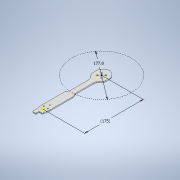
# Autodesk Inventor part: Kauri arm long
Saved by Autodesk Inventor 2020 (Build 240168000, 168)
## iProperties
Created: 2022-04-26
Part Number: Kauri arm long
Material: Generic
Document SubType Name: Modeling
Designer: Steve3
Density: 1 g/cm^3
Appearance: Default
Mass: 28.618 g
Surface Area: 128.182 cm^2
Volume: 28.618 cm^3
Sending System: Autodesk Inventor 2020
Preprocessor: ST-DEVELOPER v18
Title: Y:\Street League\Frames\Kauri\AAA LeadFingers version 2\github files\Kauri arm.stp
Author: Steven
Autodesk Inventor part; units mm, degrees
ref_plane "YZ Plane" through (0, 0, 0) normal (1, 0, 0) x (0, 1, 0)
ref_plane "XZ Plane" through (0, 0, 0) normal (0, 1, 0) x (-1, 0, 0)
ref_plane "XY Plane" through (0, 0, 0) normal (0, 0, 1) x (1, 0, 0)
sketch "Sketch3" plane through (0, 0, 0) normal (0, 1, 0) x (-1, 0, 0)
  line L0 (6.6262, -36.1747) -> (16.6262, -27.3275)
  arc A0 (16.6262, -27.3275) -> (20, -19.8379) centre (10, -19.8379) ccw
  line L1 (20, -19.8379) -> (20, -7.6759)
  arc A1 (20, -7.6759) -> (18, -1.6759) centre (10, -7.6759) ccw
  line L2 (18, -1.6759) -> (14.5, 2.9908)
  arc A2 (12.5, 8.9908) -> (14.5, 2.9908) centre (22.5, 8.9908) ccw
  arc A3 (-14.5, 2.9908) -> (-12.5, 8.9908) centre (-22.5, 8.9908) ccw
  line L3 (-14.5, 2.9908) -> (-18, -1.6759)
  arc A4 (-18, -1.6759) -> (-20, -7.6759) centre (-10, -7.6759) ccw
  line L4 (-20, -7.6759) -> (-20, -19.8379)
  arc A5 (-20, -19.8379) -> (-16.6262, -27.3275) centre (-10, -19.8379) ccw
  line L5 (-16.6262, -27.3275) -> (-6.6262, -36.1747)
  arc A6 (-6.6262, -36.1747) -> (6.6262, -36.1747) centre (0, -28.6852) ccw
  line L6 (-7.8135, -19.9641) -> (-6.7529, -18.9034)
  arc A7 (-4.5608, -21.0955) -> (-6.7529, -18.9034) centre (-5.6569, -19.9994) ccw
  line L7 (-4.5608, -21.0955) -> (-5.6215, -22.1561)
  arc A8 (-7.8135, -19.9641) -> (-5.6215, -22.1561) centre (-6.7175, -21.0601) ccw
  arc A9 (5.6215, -22.1561) -> (7.8135, -19.9641) centre (6.7175, -21.0601) ccw
  line L8 (5.6215, -22.1561) -> (4.5608, -21.0955)
  arc A10 (6.7529, -18.9034) -> (4.5608, -21.0955) centre (5.6569, -19.9994) ccw
  line L9 (6.7529, -18.9034) -> (7.8135, -19.9641)
  arc A11 (-6.7529, -9.7817) -> (-4.5608, -7.5897) centre (-5.6569, -8.6857) ccw
  line L10 (-6.7529, -9.7817) -> (-7.8135, -8.7211)
  arc A12 (-5.6215, -6.5291) -> (-7.8135, -8.7211) centre (-6.7175, -7.6251) ccw
  line L11 (-5.6215, -6.5291) -> (-4.5608, -7.5897)
  arc A13 (7.8135, -8.7211) -> (5.6215, -6.5291) centre (6.7175, -7.6251) ccw
  line L12 (7.8135, -8.7211) -> (6.7529, -9.7817)
  arc A14 (4.5608, -7.5897) -> (6.7529, -9.7817) centre (5.6569, -8.6857) ccw
  line L13 (4.5608, -7.5897) -> (5.6215, -6.5291)
  circle A15 centre (0, -14.3426) radius 3
  line L14 (-12.5, 8.9908) -> (12.5, 8.9908) construction
  arc A16 (12.5, 149.6916) -> (12.2297, 154.0328) centre (-22.5, 149.6916) ccw
  line L15 (12.2297, 154.0328) -> (10, 171.8706)
  line L16 (10, 171.8706) -> (10, 179.8706)
  arc A17 (10, 179.8706) -> (8, 181.8706) centre (8, 179.8706) ccw
  line L17 (8, 181.8706) -> (2, 181.8706)
  arc A18 (2, 181.8706) -> (0, 179.8706) centre (2, 179.8706) ccw
  line L18 (0, 179.8706) -> (0, 173.8706)
  arc A19 (-2, 171.8706) -> (0, 173.8706) centre (-2, 173.8706) ccw
  line L19 (-2, 171.8706) -> (-8.2344, 171.8706)
  arc A20 (-8.2344, 171.8706) -> (-10.219, 170.1187) centre (-8.2344, 169.8706) ccw
  line L20 (-10.219, 170.1187) -> (-12.2297, 154.0328)
  arc A21 (-12.2297, 154.0328) -> (-12.5, 149.6916) centre (22.5, 149.6916) ccw
  circle A22 centre (6, 151.8706) radius 1.5
  circle A23 centre (-6, 151.8706) radius 1.5
  circle A24 centre (0, 139.4442) radius 1.5
  circle A25 centre (0, 160.6574) radius 4
  line L21 (-12.5, 149.6916) -> (12.5, 149.6916) construction
  line L22 (0, -14.3426) -> (0, 160.6574) construction
  line L23 (12.5, 8.9908) -> (12.5, 149.6916)
  line L24 (-12.5, 149.6916) -> (-12.5, 8.9908)
  dimension "d4" = 21.2132
  dimension "d7" = 12
  dimension "d10" = 175
  constraints: 50 end point, 42 point on circle, 26 centre point, 2 perpendicular, 1 parallel
  measures "d4" distance of A25.centre A24.centre
  measures "d7" distance of A23.centre A22.centre
  measures "d10" distance of L22.start L22.end
extrude "Extrusion1" add sketch "Sketch3" along normal blind 3
sketch "Sketch4" plane through (0, 3, 0) normal (0, 1, 0) x (1, 0, 0)
  circle A0 centre (0, 14.3426) radius 3 construction
  circle A1 centre (0, 14.3426) radius 88.9 construction
  circle A2 centre (0, -160.6574) radius 4 projected
  point P0 (0, 0)
  dimension "d9" = 177.8
  dimension "d11" = 175
  constraints: 1 centre point, 1 coincident
  measures "d9" diameter of A1
  measures "d11" distance of A2.centre A0.centre
sketch "Sketch5" plane through (0, 3, 0) normal (0, 1, 0) x (1, 0, 0)
  line L0 (-18, 1.6759) -> (-14.5, -2.9908) projected
  arc A0 (-12.5, -8.9908) -> (-14.5, -2.9908) centre (-22.5, -8.9908) ccw projected
  line L1 (-12.5, -8.9908) -> (-12.5, -149.6916) projected
  line L2 (14.5, -2.9908) -> (18, 1.6759) projected
  arc A1 (14.5, -2.9908) -> (12.5, -8.9908) centre (22.5, -8.9908) ccw projected
  line L3 (12.5, -149.6916) -> (12.5, -8.9908) projected
  circle A2 centre (0, 14.3426) radius 3 construction
  circle A3 centre (0, -139.4442) radius 1.5 construction
  line L4 (0, 14.3426) -> (0, -139.4442) construction
  line L5 (7.5, 14.3426) -> (7.5, -139.4442)
  line L6 (-7.5, 14.3426) -> (-7.5, -139.4442)
  arc A4 (14.5, -2.9908) -> (12.5, -8.9908) centre (22.5, -8.9908) ccw projected
  line L7 (14.5, -2.9908) -> (5.7311, -14.6826)
  arc A5 (-12.5, -8.9908) -> (-14.5, -2.9908) centre (-22.5, -8.9908) ccw projected
  line L8 (-14.5, -2.9908) -> (-5.817, -14.5681)
  circle A6 centre (0, 14.3426) radius 88.9 construction
  line L9 (7.5, -74.2405) -> (12.5, -80.9071)
  line L10 (-7.5, -74.2405) -> (-12.5, -80.9071)
  point P0 (0, 0)
  point P1 (7.5, -12.3241)
  point P2 (-7.5, -12.3241)
  dimension "d12" = 7.5
  dimension "d13" = 7.5
  dimension "d14" = 143.13
  dimension "d15" = 143.13
  dimension "d16" = 143.13
  constraints: 14 end point, 4 point on line, 2 collinear, 2 parallel, 2 point on circle, 1 vertical
  measures "d12" distance between parallel lines of L4 L5
  measures "d13" distance between parallel lines of L4 L6
  measures "d14" angle of L5 L7
  measures "d15" angle of L6 L10
  measures "d16" angle of L5 L9
extrude "Extrusion2" cut sketch "Sketch5" against normal up to surface (3 mm away)
fillet "Fillet1" radius 10 5 edges at (7.5, 1.5, 12.3241) (7.5, 1.5, 74.2405) (12.5, 1.5, 80.9071) (-7.5, 1.5, 12.3241) (-7.5, 1.5, 74.2405)
body "Solid3"
